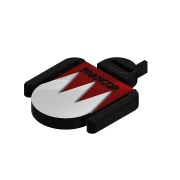
# Autodesk Inventor part: FRANCOR-MASCOT
Saved by Autodesk Inventor 2018.2 (Build 222227000, 227)
## iProperties
Manager: feesmrt
Company: FRANCOR
Part Number: FRANCOR-MASCOT
Project: Rescue Robot
Cost Center: -
Material: ABS-Kunststoff
Document SubType Name: Modeling
Designer: feesmrt
Engineer: feesmrt
Authority: feesmrt
Density: 1.06 g/cm^3
Appearance: Glänzend - schwarz
Subject: Rescue Robot
Author: feesmrt
Revision Number: 1
Autodesk Inventor part; units mm, degrees
ref_plane "YZ Plane" through (0, 0, 0) normal (1, 0, 0) x (0, 1, 0)
ref_plane "XZ Plane" through (0, 0, 0) normal (0, 1, 0) x (-1, 0, 0)
ref_plane "XY Plane" through (0, 0, 0) normal (0, 0, 1) x (1, 0, 0)
sketch "Skizze1" plane through (0, 0, 0) normal (0, 0, 1) x (1, 0, 0)
  line L0 (0, -17.5) -> (0, -17.5)
  line L1 (12.5, -5) -> (12.5, 17.5)
  line L2 (12.5, 17.5) -> (-12.5, 17.5)
  line L3 (-12.5, 17.5) -> (-12.5, -5)
  line L4 (-12.5, -17.5) -> (12.5, 17.5) construction
  line L5 (12.5, -17.5) -> (-12.5, 17.5) construction
  arc A0 (-12.5, -5) -> (0, -17.5) centre (0, -5) ccw
  arc A1 (0, -17.5) -> (12.5, -5) centre (0, -5) ccw
  line L6 (0, 145.0178) -> (0, -47.6066) construction
  line L7 (-7.5, 18.5) -> (7.5, 18.5)
  line L8 (7.5, 18.5) -> (7.5, 21)
  line L9 (0, 28.5) -> (0, 28.5)
  line L10 (-7.5, 21) -> (-7.5, 18.5)
  line L11 (-7.5, 18.5) -> (7.5, 28.5) construction
  line L12 (7.5, 18.5) -> (-7.5, 28.5) construction
  arc A2 (0, 28.5) -> (-7.5, 21) centre (0, 21) ccw
  arc A3 (7.5, 21) -> (0, 28.5) centre (0, 21) ccw
  line L13 (-5, 24.5) -> (5, 24.5)
  line L14 (5, 24.5) -> (5, 22.5)
  line L15 (5, 22.5) -> (-5, 22.5)
  line L16 (-5, 22.5) -> (-5, 24.5)
  line L17 (-5, 24.5) -> (5, 22.5) construction
  line L18 (5, 24.5) -> (-5, 22.5) construction
  line L19 (3.75, 17.5) -> (3.75, 117.5) construction
  line L20 (3, 27.8739) -> (3, 32.25)
  line L21 (3, 32.25) -> (4.5, 32.25)
  line L22 (4.5, 32.25) -> (4.5, 27)
  line L23 (-2.5, 18.5) -> (-2.5, 17.5)
  line L24 (2.5, 18.5) -> (2.5, 17.5)
  line L25 (-18, 12.5) -> (-14, 12.5)
  line L26 (-14, 12.5) -> (-14, -7.5)
  line L27 (-16, -9.5) -> (-16, -9.5)
  line L28 (-18, -7.5) -> (-18, 12.5)
  arc A4 (-12.5, 14.7913) -> (-14, 12.5) centre (-11.5, 12.5) ccw
  arc A5 (-18, -7.5) -> (-16, -9.5) centre (-16, -7.5) ccw
  arc A6 (-16, -9.5) -> (-14, -7.5) centre (-16, -7.5) ccw
  arc A7 (-12.5, 17.5) -> (-18, 12.5) centre (-12.5, 11.975) ccw
  line L29 (14, 12.5) -> (18, 12.5)
  line L30 (18, 12.5) -> (18, -7.5)
  line L31 (16, -9.5) -> (16, -9.5)
  line L32 (14, -7.5) -> (14, 12.5)
  arc A8 (14, -7.5) -> (16, -9.5) centre (16, -7.5) ccw
  arc A9 (16, -9.5) -> (18, -7.5) centre (16, -7.5) ccw
  arc A10 (14, 12.5) -> (12.5, 14.7913) centre (11.5, 12.5) ccw
  arc A11 (18, 12.5) -> (12.5, 17.5) centre (12.5, 11.975) ccw
  point P0 (0, 0)
  point P1 (0, 23.5)
  point P2 (0, 23.5)
  dimension "d0" = 25
  dimension "d1" = 35
  dimension "d2" = 12.5
  dimension "d3" = 1
  dimension "d4" = 15
  dimension "d5" = 10
  dimension "d6" = 7.5
  dimension "d7" = 2
  dimension "d8" = 10
  dimension "d9" = 4
  dimension "d10" = 100
  dimension "d11" = 3.75
  dimension "d12" = 1.5
  dimension "d13" = 3.75
  dimension "d14" = 5
  dimension "d15" = 1.5
  dimension "d16" = 5
  dimension "d17" = 4
  dimension "d18" = 2.5
  dimension "d19" = 2
  dimension "d20" = 25
  dimension "d21" = 2
  dimension "d22" = 1.5
  constraints: 64 end point, 26 point on circle, 19 tangent, 17 point on line, 12 centre point, 10 parallel, 9 perpendicular, 6 equal radius, 6 midpoint, 5 horizontal, 2 equal length, 2 horizontal alignment, 2 vertical, 2 other
  measures "d0" distance of L1.end L2.end
  measures "d1" distance of L5.start L1.end
  measures "d2" radius of A0
  measures "d3" distance between parallel lines of L7 L2
  measures "d4" distance between parallel lines of L8 L10
  measures "d5" distance between parallel lines of L7 L9
  measures "d6" radius of A2
  measures "d7" distance of L13.end L14.end
  measures "d8" distance of L14.end L15.end
  measures "d9" distance from line of L9.end L13
  measures "d10" distance of L19.start L19.end
  measures "d11" distance between parallel lines of L6 L19
  measures "d12" distance between parallel lines of L22 L20
  measures "d13" distance from line of L9.end L21
  measures "d14" distance between parallel lines of L24 L23
  measures "d15" distance between parallel lines of L3 L26
  measures "d16" distance between parallel lines of L2 L25
  measures "d17" distance between parallel lines of L26 L28
  measures "d18" radius of A4
  measures "d19" radius of A5
  measures "d20" distance from line of L2 A5.centre
  measures "d21" radius of A8
  measures "d22" distance between parallel lines of L32 L1
extrude "Extrusion2" add sketch "Skizze1" along normal blind 5
sketch "Skizze2" plane through (0, 0, 5) normal (0, 0, 1) x (1, 0, 0)
  line L0 (-12.5, 14.7913) -> (-12.5, -5) construction
  line L1 (12.5, -5) -> (12.5, 14.7913) construction
  line L2 (0, 42.2) -> (0, -27.45) construction
  line L3 (-26.3598, 0) -> (25.3933, 0) construction
  line L4 (-12.5, 10) -> (12.5, 10) construction
  line L5 (-12.5, -5) -> (12.5, -5) construction
  line L6 (12.5, 17.5) -> (2.5, 17.5) projected
  line L7 (-12.5, -5) -> (-8.3333, 10)
  line L8 (-8.3333, 10) -> (-4.1667, -5)
  line L9 (-4.1667, -5) -> (0, 10)
  line L10 (0, 10) -> (4.1667, -5)
  line L11 (4.1667, -5) -> (8.3333, 10)
  line L12 (8.3333, 10) -> (12.5, -5)
  arc A0 (-12.5, 17.5) -> (-18, 12.5) centre (-12.5, 11.975) ccw projected
  line L13 (-12.5, -5) -> (-12.5, 17.5)
  line L14 (-12.5, 17.5) -> (12.5, 17.5)
  line L15 (12.5, 17.5) -> (12.5, -5)
  point P0 (0, 0)
  dimension "d29" = 15
  constraints: 22 end point, 7 point on line, 4 equal length, 2 perpendicular, 1 collinear, 1 horizontal, 1 midpoint, 1 tangent, 1 vertical
  measures "d29" distance between parallel lines of L5 L4
extrude "Extrusion3" cut sketch "Skizze2" against normal blind 1
sketch "Skizze3" plane through (0, 0, 5) normal (0, 0, 1) x (1, 0, 0)
  line L0 (0, 42.2) -> (0, -27.45) construction
  line L1 (-7.5, 18.5) -> (-2.5, 18.5) construction
  line L2 (2.5, 18.5) -> (7.5, 18.5) construction
  line L3 (-3, 20.15) -> (1.4267, 20.15)
  arc A0 (1.4267, 20.15) -> (5, 21.8768) centre (1.4267, 24.7105) ccw
  line L4 (-3, 20.15) -> (-3, 20.3)
  line L5 (-3, 20.3) -> (1.4267, 20.3)
  line L6 (5, 21.8768) -> (7.0802, 24.5) construction
  line L7 (5, 21.8768) -> (4.8825, 21.97)
  arc A1 (1.4267, 20.3) -> (4.8825, 21.97) centre (1.3545, 24.8599) ccw
  line L8 (5, 22.5) -> (-5, 22.5) construction
  point P0 (0, 0)
  point P1 (5, 24.5)
  dimension "d32" = 3
  dimension "d33" = 0.15
  dimension "d34" = 1.4267
  dimension "d35" = 2.2
  constraints: 10 end point, 4 point on circle, 3 perpendicular, 2 centre point, 2 tangent, 2 vertical alignment, 1 equal length, 1 equal radius, 1 horizontal alignment, 1 vertical
  measures "d32" distance between parallel lines of L4 L0
  measures "d33" distance between parallel lines of L5 L3
  measures "d34" distance from line of L0 L5.end
  measures "d35" distance between parallel lines of L8 L5
extrude "Extrusion4" cut sketch "Skizze3" against normal blind 0.15
sketch "Skizze4" plane through (0, 0, 4) normal (0, 0, 1) x (1, 0, 0)
  line L0 (0, 42.2) -> (0, -27.45) construction
  line L1 (-12.5, 17.5) -> (-2.5, 17.5) construction
  line L2 (-9.5, 14.5) -> (11.7274, 14.5) construction
  line L3 (11.7274, 14.5) -> (11.7274, 11.4546) construction
  line L4 (11.7274, 11.4546) -> (-9.5, 11.4546) construction
  line L5 (-9.5, 11.4546) -> (-9.5, 14.5) construction
  line L6 (-12.5, 14.7913) -> (-12.5, 17.5) projected
  line L7 (-7.3684, 14.0752) -> (-8.7862, 14.0752)
  line L8 (-8.7862, 14.0752) -> (-8.7862, 13.2156)
  line L9 (-8.7862, 13.2156) -> (-7.4277, 13.2156)
  line L10 (-7.4277, 13.2156) -> (-7.4277, 12.855)
  line L11 (-7.4277, 12.855) -> (-8.7862, 12.855)
  line L12 (-8.7862, 12.855) -> (-8.7862, 11.3878)
  line L13 (-8.7862, 11.3878) -> (-9.1912, 11.3878)
  line L14 (-9.1912, 11.3878) -> (-9.1912, 14.4358)
  line L15 (-9.1912, 14.4358) -> (-7.3684, 14.4358)
  line L16 (-7.3684, 14.4358) -> (-7.3684, 14.0752)
  line L17 (-4.6464, 11.3878) -> (-5.1725, 11.3878)
  line L18 (-5.1725, 11.3878) -> (-6.1358, 12.6006)
  line L19 (-6.1358, 12.6006) -> (-6.6002, 12.6006)
  line L20 (-6.6002, 12.6006) -> (-6.6002, 11.3878)
  line L21 (-6.6002, 11.3878) -> (-7.0053, 11.3878)
  line L22 (-7.0053, 11.3878) -> (-7.0053, 14.4358)
  line L23 (-7.0053, 14.4358) -> (-6.2198, 14.4358)
  spline S0 degree 2 poles (-6.2198, 14.4358) (-5.958, 14.4358) (-5.6048, 14.379) (-5.4442, 14.2752) knots 0 0 0 1 2 2 2
  spline S1 degree 2 poles (-5.4442, 14.2752) (-5.2837, 14.1715) (-5.0984, 13.8479) (-5.0984, 13.6083) knots 0 0 0 1 2 2 2
  spline S2 degree 2 poles (-5.0984, 13.6083) (-5.0984, 13.2749) (-5.4393, 12.8229) (-5.7308, 12.7142) knots 0 0 0 1 2 2 2
  line L24 (-5.7308, 12.7142) -> (-4.6464, 11.3878)
  spline S3 degree 2 poles (-5.5208, 13.5762) (-5.5208, 13.7096) (-5.6147, 13.9146) (-5.7135, 13.9813) knots 0 0 0 1 2 2 2
  spline S4 degree 2 poles (-5.7135, 13.9813) (-5.7999, 14.0381) (-6.0296, 14.085) (-6.1976, 14.085) knots 0 0 0 1 2 2 2
  line L25 (-6.1976, 14.085) -> (-6.6002, 14.085)
  line L26 (-6.6002, 14.085) -> (-6.6002, 12.9389)
  line L27 (-6.6002, 12.9389) -> (-6.2445, 12.9389)
  spline S5 degree 2 poles (-6.2445, 12.9389) (-6.0691, 12.9389) (-5.79, 13.0007) (-5.6937, 13.097) knots 0 0 0 1 2 2 2
  spline S6 degree 2 poles (-5.6937, 13.097) (-5.6048, 13.181) (-5.5208, 13.4181) (-5.5208, 13.5762) knots 0 0 0 1 2 2 2
  line L28 (-4.7329, 11.3878) -> (-3.7053, 14.4358)
  line L29 (-3.7053, 14.4358) -> (-3.2064, 14.4358)
  line L30 (-3.2064, 14.4358) -> (-2.1789, 11.3878)
  line L31 (-2.1789, 11.3878) -> (-2.6062, 11.3878)
  line L32 (-2.6062, 11.3878) -> (-2.8828, 12.2399)
  line L33 (-2.8828, 12.2399) -> (-4.0462, 12.2399)
  line L34 (-4.0462, 12.2399) -> (-4.3228, 11.3878)
  line L35 (-4.3228, 11.3878) -> (-4.7329, 11.3878)
  line L36 (-2.994, 12.5857) -> (-3.4658, 14.0208)
  line L37 (-3.4658, 14.0208) -> (-3.9351, 12.5857)
  line L38 (-3.9351, 12.5857) -> (-2.994, 12.5857)
  line L39 (0.2911, 11.3878) -> (-0.1633, 11.3878)
  line L40 (-0.1633, 11.3878) -> (-1.512, 14.0159)
  line L41 (-1.512, 14.0159) -> (-1.512, 11.3878)
  line L42 (-1.512, 11.3878) -> (-1.8899, 11.3878)
  line L43 (-1.8899, 11.3878) -> (-1.8899, 14.4358)
  line L44 (-1.8899, 14.4358) -> (-1.3144, 14.4358)
  line L45 (-1.3144, 14.4358) -> (-0.0868, 12.0226)
  line L46 (-0.0868, 12.0226) -> (-0.0868, 14.4358)
  line L47 (-0.0868, 14.4358) -> (0.2911, 14.4358)
  line L48 (0.2911, 14.4358) -> (0.2911, 11.3878)
  spline S7 degree 2 poles (2.0992, 11.3334) (1.8028, 11.3334) (1.3014, 11.5335) (1.1186, 11.7336) knots 0 0 0 1 2 2 2
  spline S8 degree 2 poles (1.1186, 11.7336) (0.9358, 11.9312) (0.7357, 12.524) (0.7357, 12.9093) knots 0 0 0 1 2 2 2
  spline S9 degree 2 poles (0.7357, 12.9093) (0.7357, 13.2922) (0.9309, 13.8603) (1.1161, 14.0702) knots 0 0 0 1 2 2 2
  spline S10 degree 2 poles (1.1161, 14.0702) (1.2989, 14.2752) (1.7979, 14.4901) (2.1066, 14.4901) knots 0 0 0 1 2 2 2
  spline S11 degree 2 poles (2.1066, 14.4901) (2.2597, 14.4901) (2.529, 14.4457) (2.6426, 14.4111) knots 0 0 0 1 2 2 2
  spline S12 degree 2 poles (2.6426, 14.4111) (2.7414, 14.379) (2.9464, 14.2876) (3.0477, 14.2332) knots 0 0 0 1 2 2 2
  line L49 (3.0477, 14.2332) -> (3.0477, 13.7442)
  line L50 (3.0477, 13.7442) -> (3.0156, 13.7442)
  spline S13 degree 2 poles (3.0156, 13.7442) (2.9612, 13.7936) (2.7933, 13.9319) (2.6722, 13.9986) knots 0 0 0 1 2 2 2
  spline S14 degree 2 poles (2.6722, 13.9986) (2.5561, 14.0628) (2.282, 14.1443) (2.1041, 14.1443) knots 0 0 0 1 2 2 2
  spline S15 degree 2 poles (2.1041, 14.1443) (1.909, 14.1443) (1.5607, 13.9838) (1.4298, 13.8306) knots 0 0 0 1 2 2 2
  spline S16 degree 2 poles (1.4298, 13.8306) (1.3014, 13.675) (1.1581, 13.2032) (1.1581, 12.9093) knots 0 0 0 1 2 2 2
  spline S17 degree 2 poles (1.1581, 12.9093) (1.1581, 12.5956) (1.3088, 12.1436) (1.4397, 11.988) knots 0 0 0 1 2 2 2
  spline S18 degree 2 poles (1.4397, 11.988) (1.5681, 11.8373) (1.9115, 11.6842) (2.1041, 11.6842) knots 0 0 0 1 2 2 2
  spline S19 degree 2 poles (2.1041, 11.6842) (2.2795, 11.6842) (2.5784, 11.7706) (2.6945, 11.8349) knots 0 0 0 1 2 2 2
  spline S20 degree 2 poles (2.6945, 11.8349) (2.8056, 11.8991) (2.9711, 12.0325) (3.018, 12.0794) knots 0 0 0 1 2 2 2
  line L51 (3.018, 12.0794) -> (3.0477, 12.0794)
  line L52 (3.0477, 12.0794) -> (3.0477, 11.5953)
  spline S21 degree 2 poles (3.0477, 11.5953) (2.9464, 11.5483) (2.7686, 11.4619) (2.6426, 11.4224) knots 0 0 0 1 2 2 2
  spline S22 degree 2 poles (2.6426, 11.4224) (2.5092, 11.3779) (2.282, 11.3334) (2.0992, 11.3334) knots 0 0 0 1 2 2 2
  spline S23 degree 2 poles (5.5819, 14.0875) (5.7548, 13.885) (5.9475, 13.2922) (5.9475, 12.9118) knots 0 0 0 1 2 2 2
  spline S24 degree 2 poles (5.9475, 12.9118) (5.9475, 12.5413) (5.7598, 11.9411) (5.5819, 11.7385) knots 0 0 0 1 2 2 2
  spline S25 degree 2 poles (5.5819, 11.7385) (5.3942, 11.5261) (4.8977, 11.3236) (4.5989, 11.3236) knots 0 0 0 1 2 2 2
  spline S26 degree 2 poles (4.5989, 11.3236) (4.2901, 11.3236) (3.7961, 11.5335) (3.6158, 11.7385) knots 0 0 0 1 2 2 2
  spline S27 degree 2 poles (3.6158, 11.7385) (3.4404, 11.9411) (3.2527, 12.5363) (3.2527, 12.9118) knots 0 0 0 1 2 2 2
  spline S28 degree 2 poles (3.2527, 12.9118) (3.2527, 13.2946) (3.4429, 13.8776) (3.6183, 14.0875) knots 0 0 0 1 2 2 2
  spline S29 degree 2 poles (3.6183, 14.0875) (3.7961, 14.29) (4.2926, 14.5) (4.5989, 14.5) knots 0 0 0 1 2 2 2
  spline S30 degree 2 poles (4.5989, 14.5) (4.9101, 14.5) (5.409, 14.2826) (5.5819, 14.0875) knots 0 0 0 1 2 2 2
  spline S31 degree 2 poles (5.5251, 12.9118) (5.5251, 13.2131) (5.3942, 13.68) (5.2756, 13.8331) knots 0 0 0 1 2 2 2
  spline S32 degree 2 poles (5.2756, 13.8331) (5.1546, 13.9912) (4.8137, 14.1493) (4.6013, 14.1493) knots 0 0 0 1 2 2 2
  spline S33 degree 2 poles (4.6013, 14.1493) (4.3815, 14.1493) (4.0505, 13.9961) (3.9245, 13.8331) knots 0 0 0 1 2 2 2
  spline S34 degree 2 poles (3.9245, 13.8331) (3.8035, 13.6775) (3.6751, 13.2082) (3.6751, 12.9118) knots 0 0 0 1 2 2 2
  spline S35 degree 2 poles (3.6751, 12.9118) (3.6751, 12.3116) (4.1789, 11.6743) (4.6013, 11.6743) knots 0 0 0 1 2 2 2
  spline S36 degree 2 poles (4.6013, 11.6743) (5.0237, 11.6743) (5.5251, 12.3116) (5.5251, 12.9118) knots 0 0 0 1 2 2 2
  line L53 (8.7509, 11.3878) -> (8.2248, 11.3878)
  line L54 (8.2248, 11.3878) -> (7.2615, 12.6006)
  line L55 (7.2615, 12.6006) -> (6.7972, 12.6006)
  line L56 (6.7972, 12.6006) -> (6.7972, 11.3878)
  line L57 (6.7972, 11.3878) -> (6.3921, 11.3878)
  line L58 (6.3921, 11.3878) -> (6.3921, 14.4358)
  line L59 (6.3921, 14.4358) -> (7.1775, 14.4358)
  spline S37 degree 2 poles (7.1775, 14.4358) (7.4394, 14.4358) (7.7926, 14.379) (7.9531, 14.2752) knots 0 0 0 1 2 2 2
  spline S38 degree 2 poles (7.9531, 14.2752) (8.1137, 14.1715) (8.2989, 13.8479) (8.2989, 13.6083) knots 0 0 0 1 2 2 2
  spline S39 degree 2 poles (8.2989, 13.6083) (8.2989, 13.2749) (7.9581, 12.8229) (7.6666, 12.7142) knots 0 0 0 1 2 2 2
  line L60 (7.6666, 12.7142) -> (8.7509, 11.3878)
  spline S40 degree 2 poles (7.8766, 13.5762) (7.8766, 13.7096) (7.7827, 13.9146) (7.6839, 13.9813) knots 0 0 0 1 2 2 2
  spline S41 degree 2 poles (7.6839, 13.9813) (7.5975, 14.0381) (7.3677, 14.085) (7.1998, 14.085) knots 0 0 0 1 2 2 2
  line L61 (7.1998, 14.085) -> (6.7972, 14.085)
  line L62 (6.7972, 14.085) -> (6.7972, 12.9389)
  line L63 (6.7972, 12.9389) -> (7.1528, 12.9389)
  spline S42 degree 2 poles (7.1528, 12.9389) (7.3282, 12.9389) (7.6073, 13.0007) (7.7037, 13.097) knots 0 0 0 1 2 2 2
  spline S43 degree 2 poles (7.7037, 13.097) (7.7926, 13.181) (7.8766, 13.4181) (7.8766, 13.5762) knots 0 0 0 1 2 2 2
  point P0 (0, 0)
  dimension "d0" = 25
  dimension "d38" = 3
  dimension "d39" = 3
  constraints: 2 other
  measures "d38" distance from line of L6 L2.start
  measures "d39" distance from line of L1 L2.start
extrude "Extrusion5" add sketch "Skizze4" along normal blind 0.5
chamfer "Fase1" distance 1 angle 45 2 edges at (-12.5, 16.1456, 5) (12.5, 16.1456, 5)
chamfer "Fase2" distance 1 angle 45 1 edges at (0, 17.5, 5)
fillet "Rundung1" radius 1 10 edges at (-13.8716, 13.291, 5) (-16, -9.5, 5) (-18, 2.5, 5) (-14, 2.5, 5) (16, -9.5, 5) (18, 2.5, 5) (13.8716, 13.291, 5) (14, 2.5, 5) (-16.5725, 15.7087, 5) (16.5725, 15.7087, 5)
fillet "Rundung2" radius 0.25 6 edges at (-7.5, 19.75, 5) (6.7082, 24.3541, 5) (7.5, 19.75, 5) (3, 30.0619, 5) (4.5, 29.625, 5) (3.75, 32.25, 5)
equation "\"d2\" = 0.5 * d0"
equation "\"d3\" = 0.1 * d5"
equation "\"d6\" = 0.5 * d4"
equation "\"d7\" = 0.2 * d8"
equation "\"d8\" = 0.666667 * d4"
equation "\"d9\" = 0.4 * d5"
equation "\"d11\" = 0.25 * d4"
equation "\"d12\" = 0.1 * d4"
equation "\"d13\" = 0.25 * d4"
equation "\"d14\" = 0.333333 * d4"
equation "\"d19\" = 0.5 * d17"
equation "\"d21\" = d19"
equation "\"d22\" = d15"
